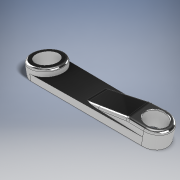
# Autodesk Inventor part: INTROWRENCH
Saved by Autodesk Inventor 2019 (Build 230136000, 136)
## iProperties
Created: 2020-05-24
Part Number: INTROWRENCH
Material: Generic
Document SubType Name: Modeling
Designer: Manoj
Density: 1 g/cm^3
Appearance: Chrome - Polished
Author: Manoj
Autodesk Inventor part; units mm, degrees
ref_plane "YZ Plane" through (0, 0, 0) normal (1, 0, 0) x (0, 1, 0)
ref_plane "XZ Plane" through (0, 0, 0) normal (0, 1, 0) x (-1, 0, 0)
ref_plane "XY Plane" through (0, 0, 0) normal (0, 0, 1) x (1, 0, 0)
sketch "Sketch4" plane through (0, 0, 0) normal (0, 1, 0) x (-1, 0, 0)
  arc A0 (21.1505, -7.4517) -> (21.1505, 7.4517) centre (22, 0) ccw
  line L0 (0, -10.9408) -> (0, 10.83) construction
  arc A1 (-22, 5) -> (-22, -5) centre (-22, 0) ccw
  line L1 (22, -7.5) -> (-22, -5)
  line L2 (22, 7.5) -> (-22, 5)
  point P0 (0, 0)
  dimension "d14" = 15
  dimension "d16" = 22
  dimension "d17" = 22
  constraints: 6 end point, 6 point on circle, 2 centre point, 2 point on line, 1 vertical
  measures "d14" diameter of A0
  measures "d16" distance of point (0, 0) A0.centre
  measures "d17" distance of A1.centre point (0, 0)
extrude "Extrusion3" add sketch "Sketch4" along normal blind 3 contours L1 A1 L2 A0
sketch "Sketch5" plane through (0, 3, 0) normal (0, 1, 0) x (1, 0, 0)
  line L0 (0, 0) -> (-22, 0) construction
  circle A0 centre (-22, 0) radius 7.5
  line L1 (0, 0) -> (22, 0) construction
  circle A1 centre (22, 0) radius 5
  dimension "d20" = 22
  dimension "d21" = 15
  dimension "d22" = 22
  dimension "d23" = 10
  constraints: 4 end point, 2 centre point, 2 coincident, 2 horizontal
  measures "d20" distance of L0.start L0.end
  measures "d21" diameter of A0
  measures "d22" distance of L0.start L1.end
  measures "d23" diameter of A1
extrude "Extrusion4" add sketch "Sketch5" along normal blind 3
sketch "Sketch6" plane through (-22, 6, 0) normal (0, 1, 0) x (1, 0, 0)
  circle A0 centre (0, 0) radius 5
  point P0 (22, 0)
  dimension "d26" = 10
  constraints: 1 centre point
  measures "d26" diameter of A0
extrude "Extrusion5" cut sketch "Sketch6" against normal blind 10.9375
sketch "Sketch7" plane through (22, 6, 0) normal (0, 1, 0) x (1, 0, 0)
  circle A0 centre (0, 0) radius 3.5
  point P0 (-22, 0)
  dimension "d29" = 7
  constraints: 1 centre point
  measures "d29" diameter of A0
extrude "Extrusion6" cut sketch "Sketch7" against normal blind 10.9375
sketch "Sketch8" plane through (0, 0, 0) normal (0, 0, 1) x (1, 0, 0)
  line L0 (27, 6) -> (17, 6) projected
  line L1 (22, 0) -> (22, 0) projected
  line L2 (22, 0) -> (22, 3) projected
  line L3 (22, 3) -> (22, 3) projected
  line L4 (22, 0) -> (22, 3) projected
  line L5 (18.5, 6) -> (25.5, 6) projected
  line L6 (22, 0) -> (22, 3) projected
  line L7 (22, 6) -> (22, 3)
  line L8 (22, 3) -> (2, 3)
  line L9 (-21.1505, 3) -> (22, 3) projected
  line L10 (2, 3) -> (17, 6)
  line L11 (27, 6) -> (17, 6) projected
  line L12 (17, 6) -> (22, 6)
  point P0 (0, 0)
  dimension "d32" = 20
  constraints: 8 end point, 1 collinear, 1 midpoint, 1 perpendicular, 1 point on line
  measures "d32" distance of L2.end L8.end
extrude "Extrusion7" add sketch "Sketch8" along normal mid plane 10
delete faces "Delete1" heal yes whole lump no faces at (20.9091, 3, 0.4137) (22, 4, -1.1667)
fillet "Fillet1" radius 5 1 edges at (17, 6, 0)
fillet "Fillet2" radius 5 1 edges at (2, 3, 0)
fillet "Fillet3" radius 1 1 edges at (-29.5, 6, 0)
fillet "Fillet4" radius 1 9 edges at (17.0024, 5.9757, 5) (9.5, 4.5, 5) (1.9976, 3.0243, 5) (27, 6, 0) (19.7475, 6, -5) (17.0024, 5.9757, -5) (9.5, 4.5, -5) (1.9976, 3.0243, -5) (19.7475, 6, 5)
fillet "Fillet5" radius 0.3 1 edges at (18.5, 6, 0)
body "Solid2"
